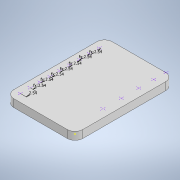
# Autodesk Inventor part: Część3
Saved by Autodesk Inventor 2020.3 (Build 243373000, 373)
## iProperties
Created: 2021-03-18
Part Number: Część3
Material: Ogólny
Document SubType Name: Modeling
Designer: patry
Density: 1 g/cm^3
Appearance: Domyślna
Author: patry
Autodesk Inventor part; units mm, degrees
ref_plane "YZ Plane" through (0, 0, 0) normal (1, 0, 0) x (0, 1, 0)
ref_plane "XZ Plane" through (0, 0, 0) normal (0, 1, 0) x (-1, 0, 0)
ref_plane "XY Plane" through (0, 0, 0) normal (0, 0, 1) x (1, 0, 0)
sketch "Szkic1" plane through (0, 0, 0) normal (0, 1, 0) x (-1, 0, 0)
  line L0 (2, 0) -> (15.8, 0)
  line L1 (17.8, -2) -> (17.8, -23.4)
  line L2 (15.8, -25.4) -> (2, -25.4)
  line L3 (0, -23.4) -> (0, -2)
  arc A0 (17.8, -2) -> (15.8, 0) centre (15.8, -2) ccw
  arc A1 (15.8, -25.4) -> (17.8, -23.4) centre (15.8, -23.4) ccw
  arc A2 (0, -23.4) -> (2, -25.4) centre (2, -23.4) ccw
  arc A3 (2, 0) -> (0, -2) centre (2, -2) ccw
  point P0 (0, 0)
  point P1 (17.8, -25.4)
  point P2 (17.8, 0)
  point P3 (0, -25.4)
  dimension "d0" = 17.8
  dimension "d1" = 25.4
  dimension "d2" = 2
  constraints: 8 end point, 8 point on circle, 8 point on line, 8 tangent, 4 centre point, 3 equal radius, 2 parallel, 1 horizontal, 1 perpendicular
  measures "d0" distance of point (17.8, -25.4) point (0, -25.4)
  measures "d1" distance of point (17.8, 0) point (17.8, -25.4)
  measures "d2" radius of A0
extrude "Wyciągnięcie proste1" add sketch "Szkic1" along normal blind 2
sketch "Szkic2" plane through (0, 2, 0) normal (0, 1, 0) x (1, 0, 0)
  point P0 (0, 0)
  point P1 (-2.019, 9.2156)
  point P2 (-2.019, 13.97)
  point P3 (-2.019, 18.4638)
  point P4 (-2.019, 22.3064)
  point P5 (-2.019, 25.4977)
  point P6 (-16.067, 1.9937)
  point P7 (-16.067, 4.5337)
  point P8 (-16.067, 7.0737)
  point P9 (-16.067, 9.6137)
  point P10 (-16.067, 12.1537)
  point P11 (-16.067, 14.6937)
  point P12 (-16.067, 17.2337)
  point P13 (-16.067, 19.7737)
  point P14 (-16.067, 22.3137)
  dimension "d5" = 2.54
  dimension "d6" = 2.54
  dimension "d7" = 2.54
  dimension "d8" = 2.54
  dimension "d9" = 2.54
  dimension "d10" = 2.54
  dimension "d11" = 2.54
  dimension "d12" = 2.54
  constraints: 8 vertical alignment
  measures "d5" distance of point (-16.067, 4.534) point (-16.067, 1.994)
  measures "d6" distance of point (-16.067, 7.074) point (-16.067, 4.534)
  measures "d7" distance of point (-16.067, 9.614) point (-16.067, 7.074)
  measures "d8" distance of point (-16.067, 12.154) point (-16.067, 9.614)
  measures "d9" distance of point (-16.067, 14.694) point (-16.067, 12.154)
  measures "d10" distance of point (-16.067, 17.234) point (-16.067, 14.694)
  measures "d11" distance of point (-16.067, 19.774) point (-16.067, 17.234)
  measures "d12" distance of point (-16.067, 22.314) point (-16.067, 19.774)
equation "\"d6\" = d5"
equation "\"d7\" = d6"
equation "\"d8\" = d7"
equation "\"d9\" = d8"
equation "\"d10\" = d9"
equation "\"d11\" = d10"
equation "\"d12\" = d11"
